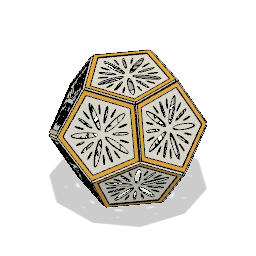
20-Day 14 - Diwali LampShade v2 (Autodesk Fusion 360 design; units mm, degrees)
Autodesk Fusion 360 part; units mm, degrees
(part 1 of 3)
sketch "Sketch1" plane through (0, 0, 0) normal (0, 1, 0) x (1, 0, 0)
  line L0 (-50, 0) -> (-15.4508, -47.5528)
  line L1 (-15.4508, -47.5528) -> (40.4508, -29.3893)
  line L2 (40.4508, -29.3893) -> (40.4508, 29.3893)
  line L3 (40.4508, 29.3893) -> (-15.4508, 47.5528)
  line L4 (-15.4508, 47.5528) -> (-50, 0)
  line L5 (-13.541, -41.675) -> (35.4508, -25.7565)
  line L6 (35.4508, -25.7565) -> (35.4508, 25.7565)
  line L7 (35.4508, 25.7565) -> (-13.541, 41.675)
  line L8 (-13.541, 41.675) -> (-43.8197, 0)
  line L9 (-43.8197, 0) -> (-13.541, -41.675)
  spline S0 degree 5 poles (-5, 0) (-5, 0.1873) (-5.1504, 0.5619) (-5.827, 1.1149) (-7.5942, 1.7986) (-11.0069, 2.4812) (-15.2799, 2.923) (-20, 3.0764) (-24.7201, 2.923) (-28.9931, 2.4812) (-32.4058, 1.7986) (-34.6148, 0.944) (-35.3821, 0) (-34.6148, -0.944) (-32.4058, -1.7986) (-28.9931, -2.4812) (-24.7201, -2.923) (-20, -3.0764) (-15.2799, -2.923) (-11.0069, -2.4812) (-7.5942, -1.7986) (-5.827, -1.1149) (-5.1504, -0.5619) (-5, -0.1873) (-5, 0) knots 0 0 0 0 0 0 0.05 0.1 0.15 0.2 0.25 0.3 0.35 0.4 0.45 0.5 0.55 0.6 0.65 0.7 0.75 0.8 0.85 0.9 0.95 1 1 1 1 1 1
  spline S1 degree 5 poles (-1.5451, -4.7553) (-1.7232, -4.6974) (-2.126, -4.7246) (-2.861, -5.1973) (-4.0573, -6.6667) (-5.7611, -9.7015) (-7.5016, -13.6288) (-9.1062, -18.0705) (-10.4188, -22.607) (-11.3191, -26.8073) (-11.7245, -30.264) (-11.5944, -32.6289) (-10.9337, -33.6504) (-9.7987, -33.2123) (-8.3034, -31.3756) (-6.5996, -28.3408) (-4.8591, -24.4135) (-3.2545, -19.9718) (-1.9418, -15.4352) (-1.0416, -11.2349) (-0.6361, -7.7783) (-0.7403, -5.8864) (-1.0571, -5.0719) (-1.3669, -4.8132) (-1.5451, -4.7553) knots 0 0 0 0 0 0 0.05 0.1 0.15 0.2 0.25 0.3 0.35 0.4 0.45 0.5 0.55 0.6 0.65 0.7 0.75 0.8 0.85 0.9 0.95 1 1 1 1 1 1
  spline S2 degree 5 poles (4.0451, -2.9389) (3.935, -3.0905) (3.8364, -3.4819) (4.0588, -4.327) (5.0866, -5.9189) (7.4464, -8.477) (10.6436, -11.346) (14.3721, -14.2446) (18.281, -16.8949) (21.9975, -19.049) (25.1597, -20.5028) (27.449, -21.1098) (28.6247, -20.7971) (28.5588, -19.5823) (27.2741, -17.5926) (24.9143, -15.0344) (21.7171, -12.1654) (17.9886, -9.2668) (14.0797, -6.6166) (10.3632, -4.4624) (7.201, -3.0086) (5.3695, -2.523) (4.497, -2.5727) (4.1552, -2.7874) (4.0451, -2.9389) knots 0 0 0 0 0 0 0.05 0.1 0.15 0.2 0.25 0.3 0.35 0.4 0.45 0.5 0.55 0.6 0.65 0.7 0.75 0.8 0.85 0.9 0.95 1 1 1 1 1 1
  spline S3 degree 5 poles (4.0451, 2.9389) (4.1552, 2.7874) (4.497, 2.5727) (5.3695, 2.523) (7.201, 3.0086) (10.3632, 4.4624) (14.0797, 6.6166) (17.9886, 9.2668) (21.7171, 12.1654) (24.9143, 15.0344) (27.2741, 17.5926) (28.5588, 19.5823) (28.6247, 20.7971) (27.449, 21.1098) (25.1597, 20.5028) (21.9975, 19.049) (18.281, 16.8949) (14.3721, 14.2446) (10.6436, 11.346) (7.4464, 8.477) (5.0866, 5.9189) (4.0588, 4.327) (3.8364, 3.4819) (3.935, 3.0905) (4.0451, 2.9389) knots 0 0 0 0 0 0 0.05 0.1 0.15 0.2 0.25 0.3 0.35 0.4 0.45 0.5 0.55 0.6 0.65 0.7 0.75 0.8 0.85 0.9 0.95 1 1 1 1 1 1
  spline S4 degree 5 poles (-1.5451, 4.7553) (-1.3669, 4.8132) (-1.0571, 5.0719) (-0.7403, 5.8864) (-0.6361, 7.7783) (-1.0416, 11.2349) (-1.9418, 15.4352) (-3.2545, 19.9718) (-4.8591, 24.4135) (-6.5996, 28.3408) (-8.3034, 31.3756) (-9.7987, 33.2123) (-10.9337, 33.6504) (-11.5944, 32.6289) (-11.7245, 30.264) (-11.3191, 26.8073) (-10.4188, 22.607) (-9.1062, 18.0705) (-7.5016, 13.6288) (-5.7611, 9.7015) (-4.0573, 6.6667) (-2.861, 5.1973) (-2.126, 4.7246) (-1.7232, 4.6974) (-1.5451, 4.7553) knots 0 0 0 0 0 0 0.05 0.1 0.15 0.2 0.25 0.3 0.35 0.4 0.45 0.5 0.55 0.6 0.65 0.7 0.75 0.8 0.85 0.9 0.95 1 1 1 1 1 1
  spline S5 degree 5 poles (-10, 7.2654) (-9.946, 7.3337) (-9.9164, 7.5257) (-10.1101, 7.9769) (-10.8326, 8.8775) (-12.3971, 10.3808) (-14.4507, 12.1067) (-16.7835, 13.883) (-19.1692, 15.538) (-21.3871, 16.9176) (-23.2347, 17.8934) (-24.5416, 18.3712) (-25.1825, 18.2995) (-25.0928, 17.6796) (-24.2842, 16.5762) (-22.8328, 15.1015) (-20.8692, 13.4003) (-18.5684, 11.6352) (-16.1427, 9.973) (-13.8307, 8.571) (-11.8705, 7.5662) (-10.7531, 7.1642) (-10.2405, 7.1161) (-10.054, 7.1972) (-10, 7.2654) knots 0 0 0 0 0 0 0.05 0.1 0.15 0.2 0.25 0.3 0.35 0.4 0.45 0.5 0.55 0.6 0.65 0.7 0.75 0.8 0.85 0.9 0.95 1 1 1 1 1 1
  line L10 (-25, 17.7501) -> (-25, 18.1636)
  spline S6 degree 5 poles (-10, -7.2654) (-10.0482, -7.193) (-10.2217, -7.1055) (-10.7106, -7.1503) (-11.7904, -7.5591) (-13.7037, -8.5825) (-15.9796, -10.0023) (-18.3899, -11.672) (-20.7012, -13.4295) (-22.6985, -15.1125) (-24.1976, -16.5682) (-25.0558, -17.6634) (-25.1857, -18.2951) (-24.5684, -18.4014) (-23.2691, -17.9733) (-21.4181, -17.0487) (-19.1933, -15.7069) (-16.8037, -14.0642) (-14.4732, -12.2708) (-12.4254, -10.5052) (-10.864, -8.9514) (-10.1364, -8.013) (-9.9323, -7.5403) (-9.9518, -7.3379) (-10, -7.2654) knots 0 0 0 0 0 0 0.05 0.1 0.15 0.2 0.25 0.3 0.35 0.4 0.45 0.5 0.55 0.6 0.65 0.7 0.75 0.8 0.85 0.9 0.95 1 1 1 1 1 1
  spline S7 degree 5 poles (3.8197, -11.7557) (3.7358, -11.7792) (3.5991, -11.9171) (3.4905, -12.396) (3.5457, -13.5492) (3.9278, -15.6851) (4.5748, -18.2884) (5.4179, -21.0967) (6.3752, -23.8379) (7.3586, -26.2576) (8.2798, -28.1331) (9.0562, -29.2878) (9.6169, -29.6065) (9.9087, -29.0523) (9.9031, -27.6843) (9.5957, -25.6382) (9.0071, -23.1077) (8.1832, -20.3273) (7.1977, -17.5567) (6.1514, -15.0636) (5.1561, -13.0984) (4.4885, -12.1165) (4.102, -11.7763) (3.9035, -11.7322) (3.8197, -11.7557) knots 0 0 0 0 0 0 0.05 0.1 0.15 0.2 0.25 0.3 0.35 0.4 0.45 0.5 0.55 0.6 0.65 0.7 0.75 0.8 0.85 0.9 0.95 1 1 1 1 1 1
  spline S8 degree 5 poles (12.3607, 0) (12.3571, -0.087) (12.4461, -0.2597) (12.8679, -0.5109) (13.9818, -0.8148) (16.1312, -1.1114) (18.807, -1.3006) (21.7384, -1.3665) (24.6413, -1.3031) (27.2464, -1.1156) (29.3148, -0.819) (30.6529, -0.4374) (31.1293, -0.0027) (30.6923, 0.4461) (29.3895, 0.8635) (27.3486, 1.2034) (24.76, 1.4256) (21.8612, 1.5012) (18.9217, 1.4201) (16.2272, 1.1955) (14.0507, 0.8561) (12.9105, 0.5246) (12.4675, 0.2622) (12.3643, 0.087) (12.3607, 0) knots 0 0 0 0 0 0 0.05 0.1 0.15 0.2 0.25 0.3 0.35 0.4 0.45 0.5 0.55 0.6 0.65 0.7 0.75 0.8 0.85 0.9 0.95 1 1 1 1 1 1
  spline S9 degree 5 poles (3.8197, 11.7557) (3.9013, 11.7254) (4.093, 11.7567) (4.4623, 12.0802) (5.0955, 13.0457) (6.0418, 14.9982) (7.0486, 17.4846) (8.0171, 20.2521) (8.8539, 23.0326) (9.4806, 25.5681) (9.8377, 27.6269) (9.8883, 29.0174) (9.622, 29.6049) (9.0602, 29.328) (8.2607, 28.2179) (7.3067, 26.3819) (6.2955, 23.9887) (5.3278, 21.2551) (4.4965, 18.4344) (3.8775, 15.8024) (3.5277, 13.6276) (3.4906, 12.4407) (3.6033, 11.9383) (3.738, 11.786) (3.8197, 11.7557) knots 0 0 0 0 0 0 0.05 0.1 0.15 0.2 0.25 0.3 0.35 0.4 0.45 0.5 0.55 0.6 0.65 0.7 0.75 0.8 0.85 0.9 0.95 1 1 1 1 1 1
  line L11 (0, 0) -> (32.2957, 0) construction
  line L12 (-20, 1) -> (-20, 3)
  spline S10 degree 5 poles (-20, 6.4984) (-19.9899, 6.5417) (-20.0193, 6.6469) (-20.2127, 6.8586) (-20.7593, 7.2342) (-21.8513, 7.8023) (-23.2443, 8.4014) (-24.806, 8.9632) (-26.3896, 9.4283) (-27.8444, 9.7572) (-29.0275, 9.9285) (-29.8175, 9.9359) (-30.1281, 9.7856) (-29.9216, 9.4946) (-29.2253, 9.0882) (-28.1165, 8.5994) (-26.7091, 8.0666) (-25.1409, 7.5331) (-23.5615, 7.0456) (-22.1199, 6.6533) (-20.9537, 6.4023) (-20.3331, 6.3432) (-20.08, 6.3871) (-20.0101, 6.4551) (-20, 6.4984) knots 0 0 0 0 0 0 0.05 0.1 0.15 0.2 0.25 0.3 0.35 0.4 0.45 0.5 0.55 0.6 0.65 0.7 0.75 0.8 0.85 0.9 0.95 1 1 1 1 1 1
  spline S11 degree 5 poles (-12.3607, 17.013) (-12.3987, 16.99) (-12.5079, 16.9855) (-12.769, 17.104) (-13.2951, 17.5078) (-14.1729, 18.3708) (-15.1731, 19.5105) (-16.19, 20.8221) (-17.1217, 22.1845) (-17.884, 23.4664) (-18.4126, 24.5387) (-18.6637, 25.2878) (-18.6168, 25.6296) (-18.2761, 25.5232) (-17.6745, 24.9865) (-16.867, 24.083) (-15.9253, 22.9091) (-14.9334, 21.5826) (-13.9816, 20.2311) (-13.1631, 18.9813) (-12.564, 17.9497) (-12.316, 17.3778) (-12.2796, 17.1234) (-12.3226, 17.036) (-12.3607, 17.013) knots 0 0 0 0 0 0 0.05 0.1 0.15 0.2 0.25 0.3 0.35 0.4 0.45 0.5 0.55 0.6 0.65 0.7 0.75 0.8 0.85 0.9 0.95 1 1 1 1 1 1
  line L13 (-20.0391, 6.3312) -> (-19.9609, 6.6656)
  line L14 (-12.2137, 17.1018) -> (-12.5076, 16.9242)
  line L15 (-30, 9.7063) -> (-30, 9.7476)
  spline S12 degree 5 poles (-12.3607, -17.013) (-12.3987, -16.99) (-12.5079, -16.9855) (-12.769, -17.104) (-13.2951, -17.5078) (-14.1729, -18.3708) (-15.1731, -19.5105) (-16.19, -20.8221) (-17.1217, -22.1845) (-17.884, -23.4664) (-18.4126, -24.5387) (-18.6637, -25.2878) (-18.6168, -25.6296) (-18.2761, -25.5232) (-17.6745, -24.9865) (-16.867, -24.083) (-15.9253, -22.9091) (-14.9334, -21.5826) (-13.9816, -20.2311) (-13.1631, -18.9813) (-12.564, -17.9497) (-12.316, -17.3778) (-12.2796, -17.1234) (-12.3226, -17.036) (-12.3607, -17.013) knots 0 0 0 0 0 0 0.05 0.1 0.15 0.2 0.25 0.3 0.35 0.4 0.45 0.5 0.55 0.6 0.65 0.7 0.75 0.8 0.85 0.9 0.95 1 1 1 1 1 1
  spline S13 degree 5 poles (-20, -6.4984) (-19.9899, -6.5417) (-20.0193, -6.6469) (-20.2127, -6.8586) (-20.7593, -7.2342) (-21.8513, -7.8023) (-23.2443, -8.4014) (-24.806, -8.9632) (-26.3896, -9.4283) (-27.8444, -9.7572) (-29.0275, -9.9285) (-29.8175, -9.9359) (-30.1281, -9.7856) (-29.9216, -9.4946) (-29.2253, -9.0882) (-28.1165, -8.5994) (-26.7091, -8.0666) (-25.1409, -7.5331) (-23.5615, -7.0456) (-22.1199, -6.6533) (-20.9537, -6.4023) (-20.3331, -6.3432) (-20.08, -6.3871) (-20.0101, -6.4551) (-20, -6.4984) knots 0 0 0 0 0 0 0.05 0.1 0.15 0.2 0.25 0.3 0.35 0.4 0.45 0.5 0.55 0.6 0.65 0.7 0.75 0.8 0.85 0.9 0.95 1 1 1 1 1 1
  spline S14 degree 5 poles (12.3607, -17.013) (12.3271, -17.0421) (12.289, -17.1445) (12.321, -17.4295) (12.5425, -18.0546) (13.092, -19.1561) (13.8668, -20.4596) (14.8, -21.8319) (15.8079, -23.1391) (16.7914, -24.2602) (17.6479, -25.0943) (18.2827, -25.5646) (18.6223, -25.6256) (18.6264, -25.2688) (18.3019, -24.5307) (17.6921, -23.4835) (16.8667, -22.2252) (15.9116, -20.8719) (14.9204, -19.5491) (13.9846, -18.3844) (13.1887, -17.4958) (12.7214, -17.0832) (12.4908, -16.97) (12.3943, -16.9839) (12.3607, -17.013) knots 0 0 0 0 0 0 0.05 0.1 0.15 0.2 0.25 0.3 0.35 0.4 0.45 0.5 0.55 0.6 0.65 0.7 0.75 0.8 0.85 0.9 0.95 1 1 1 1 1 1
  spline S15 degree 5 poles (0, -21.0292) (0.0443, -21.033) (0.1353, -21.0935) (0.2769, -21.3429) (0.4652, -21.9788) (0.668, -23.1929) (0.8073, -24.7028) (0.859, -26.3617) (0.812, -28.0115) (0.6753, -29.4967) (0.4726, -30.6748) (0.2355, -31.4285) (-0.0034, -31.6774) (-0.2164, -31.3911) (-0.3877, -30.6034) (-0.51, -29.3977) (-0.5818, -27.8946) (-0.6046, -26.2383) (-0.5802, -24.5855) (-0.5077, -23.0932) (-0.3861, -21.9065) (-0.2506, -21.2981) (-0.1305, -21.0709) (-0.0443, -21.0255) (0, -21.0292) knots 0 0 0 0 0 0 0.05 0.1 0.15 0.2 0.25 0.3 0.35 0.4 0.45 0.5 0.55 0.6 0.65 0.7 0.75 0.8 0.85 0.9 0.95 1 1 1 1 1 1
  spline S16 degree 5 poles (20, 6.4984) (20.0173, 6.4574) (20.1029, 6.3896) (20.3838, 6.332) (21.0468, 6.3494) (22.2642, 6.5317) (23.7433, 6.8658) (25.3369, 7.3292) (26.8915, 7.8838) (28.2617, 8.4728) (29.3196, 9.0296) (29.9631, 9.488) (30.126, 9.7921) (29.7879, 9.9062) (28.9857, 9.8257) (27.8013, 9.5694) (26.3495, 9.1732) (24.7673, 8.6831) (23.2029, 8.1491) (21.8061, 7.6191) (20.715, 7.1367) (20.1783, 6.8198) (19.9993, 6.6354) (19.9827, 6.5394) (20, 6.4984) knots 0 0 0 0 0 0 0.05 0.1 0.15 0.2 0.25 0.3 0.35 0.4 0.45 0.5 0.55 0.6 0.65 0.7 0.75 0.8 0.85 0.9 0.95 1 1 1 1 1 1
  spline S17 degree 5 poles (20, -6.4984) (20.0173, -6.4574) (20.1029, -6.3896) (20.3838, -6.332) (21.0468, -6.3494) (22.2642, -6.5317) (23.7433, -6.8658) (25.3369, -7.3292) (26.8915, -7.8838) (28.2617, -8.4728) (29.3196, -9.0296) (29.9631, -9.488) (30.126, -9.7921) (29.7879, -9.9062) (28.9857, -9.8257) (27.8013, -9.5694) (26.3495, -9.1732) (24.7673, -8.6831) (23.2029, -8.1491) (21.8061, -7.6191) (20.715, -7.1367) (20.1783, -6.8198) (19.9993, -6.6354) (19.9827, -6.5394) (20, -6.4984) knots 0 0 0 0 0 0 0.05 0.1 0.15 0.2 0.25 0.3 0.35 0.4 0.45 0.5 0.55 0.6 0.65 0.7 0.75 0.8 0.85 0.9 0.95 1 1 1 1 1 1
  spline S18 degree 5 poles (0, 21.0292) (0.0443, 21.033) (0.1353, 21.0935) (0.2769, 21.3429) (0.4652, 21.9788) (0.668, 23.1929) (0.8073, 24.7028) (0.859, 26.3617) (0.812, 28.0115) (0.6753, 29.4967) (0.4726, 30.6748) (0.2355, 31.4285) (-0.0034, 31.6774) (-0.2164, 31.3911) (-0.3877, 30.6034) (-0.51, 29.3977) (-0.5818, 27.8946) (-0.6046, 26.2383) (-0.5802, 24.5855) (-0.5077, 23.0932) (-0.3861, 21.9065) (-0.2506, 21.2981) (-0.1305, 21.0709) (-0.0443, 21.0255) (0, 21.0292) knots 0 0 0 0 0 0 0.05 0.1 0.15 0.2 0.25 0.3 0.35 0.4 0.45 0.5 0.55 0.6 0.65 0.7 0.75 0.8 0.85 0.9 0.95 1 1 1 1 1 1
  spline S19 degree 5 poles (12.3607, 17.013) (12.3271, 17.0421) (12.289, 17.1445) (12.321, 17.4295) (12.5425, 18.0546) (13.092, 19.1561) (13.8668, 20.4596) (14.8, 21.8319) (15.8079, 23.1391) (16.7914, 24.2602) (17.6479, 25.0943) (18.2827, 25.5646) (18.6223, 25.6256) (18.6264, 25.2688) (18.3019, 24.5307) (17.6921, 23.4835) (16.8667, 22.2252) (15.9116, 20.8719) (14.9204, 19.5491) (13.9846, 18.3844) (13.1887, 17.4958) (12.7214, 17.0832) (12.4908, 16.97) (12.3943, 16.9839) (12.3607, 17.013) knots 0 0 0 0 0 0 0.05 0.1 0.15 0.2 0.25 0.3 0.35 0.4 0.45 0.5 0.55 0.6 0.65 0.7 0.75 0.8 0.85 0.9 0.95 1 1 1 1 1 1
  line L16 (-30, 9.7476) -> (-30.715, 9.9799)
  line L17 (6.4347, -102.4282) -> (6.459, -102.4616)
  line L18 (12.5094, -93.8428) -> (12.7692, -94.0674)
  spline S20 degree 5 poles (5, -70.4437) (4.9827, -70.4847) (4.8971, -70.5525) (4.6162, -70.6101) (3.9532, -70.5927) (2.7358, -70.4104) (1.2567, -70.0763) (-0.3369, -69.6129) (-1.8915, -69.0583) (-3.2617, -68.4693) (-4.3196, -67.9125) (-4.9631, -67.4541) (-5.126, -67.15) (-4.7879, -67.0358) (-3.9857, -67.1164) (-2.8013, -67.3727) (-1.3495, -67.7689) (0.2327, -68.259) (1.7971, -68.7929) (3.1939, -69.323) (4.285, -69.8054) (4.8217, -70.1223) (5.0007, -70.3067) (5.0173, -70.4027) (5, -70.4437) knots 0 0 0 0 0 0 0.05 0.1 0.15 0.2 0.25 0.3 0.35 0.4 0.45 0.5 0.55 0.6 0.65 0.7 0.75 0.8 0.85 0.9 0.95 1 1 1 1 1 1
  line L19 (-12.2076, -17.1055) -> (-12.5137, -16.9205)
  line L20 (5.0695, -70.2789) -> (4.9305, -70.6085)
  spline S21 degree 5 poles (12.6393, -76.9421) (12.6429, -77.0291) (12.5539, -77.2018) (12.1321, -77.453) (11.0182, -77.7569) (8.8688, -78.0535) (6.193, -78.2426) (3.2616, -78.3086) (0.3587, -78.2452) (-2.2464, -78.0577) (-4.3148, -77.7611) (-5.6529, -77.3795) (-6.1293, -76.9448) (-5.6923, -76.496) (-4.3895, -76.0786) (-2.3486, -75.7387) (0.24, -75.5165) (3.1388, -75.4409) (6.0783, -75.522) (8.7728, -75.7466) (10.9493, -76.086) (12.0895, -76.4175) (12.5325, -76.6799) (12.6357, -76.8551) (12.6393, -76.9421) knots 0 0 0 0 0 0 0.05 0.1 0.15 0.2 0.25 0.3 0.35 0.4 0.45 0.5 0.55 0.6 0.65 0.7 0.75 0.8 0.85 0.9 0.95 1 1 1 1 1 1
  line L21 (-9.8099, -7.5511) -> (-10.1901, -6.9798)
  line L22 (12.6252, -76.5992) -> (12.6534, -77.285)
  spline S22 degree 5 poles (26.5451, -72.1868) (26.3669, -72.1289) (26.0571, -71.8701) (25.7403, -71.0557) (25.6361, -69.1638) (26.0416, -65.7072) (26.9418, -61.5068) (28.2545, -56.9703) (29.8591, -52.5286) (31.5996, -48.6013) (33.3034, -45.5665) (34.7987, -43.7298) (35.9337, -43.2917) (36.5944, -44.3132) (36.7245, -46.6781) (36.3191, -50.1348) (35.4188, -54.3351) (34.1062, -58.8716) (32.5016, -63.3133) (30.7611, -67.2406) (29.0573, -70.2754) (27.861, -71.7448) (27.126, -72.2174) (26.7232, -72.2447) (26.5451, -72.1868) knots 0 0 0 0 0 0 0.05 0.1 0.15 0.2 0.25 0.3 0.35 0.4 0.45 0.5 0.55 0.6 0.65 0.7 0.75 0.8 0.85 0.9 0.95 1 1 1 1 1 1
  line L23 (4.487, -2.3307) -> (3.6032, -3.5472)
  line L24 (27.2601, -72.4191) -> (25.8301, -71.9545)
  spline S23 degree 5 poles (21.1803, -65.1864) (21.0987, -65.2167) (20.907, -65.1854) (20.5377, -64.8619) (19.9045, -63.8964) (18.9582, -61.9439) (17.9514, -59.4575) (16.9829, -56.6899) (16.1461, -53.9095) (15.5194, -51.3739) (15.1623, -49.3152) (15.1117, -47.9247) (15.378, -47.3372) (15.9398, -47.6141) (16.7393, -48.7242) (17.6933, -50.5602) (18.7045, -52.9534) (19.6722, -55.687) (20.5035, -58.5077) (21.1225, -61.1397) (21.4723, -63.3145) (21.5094, -64.5014) (21.3967, -65.0038) (21.262, -65.1561) (21.1803, -65.1864) knots 0 0 0 0 0 0 0.05 0.1 0.15 0.2 0.25 0.3 0.35 0.4 0.45 0.5 0.55 0.6 0.65 0.7 0.75 0.8 0.85 0.9 0.95 1 1 1 1 1 1
  line L25 (4.1359, -11.6671) -> (3.5034, -11.8443)
  line L26 (21.4883, -65.0722) -> (20.8724, -65.3006)
  spline S24 degree 5 poles (5, -83.4405) (4.9827, -83.3995) (4.8971, -83.3317) (4.6162, -83.2741) (3.9532, -83.2915) (2.7358, -83.4737) (1.2567, -83.8079) (-0.3369, -84.2713) (-1.8915, -84.8259) (-3.2617, -85.4149) (-4.3196, -85.9716) (-4.9631, -86.4301) (-5.126, -86.7342) (-4.7879, -86.8483) (-3.9857, -86.7678) (-2.8013, -86.5115) (-1.3495, -86.1153) (0.2327, -85.6252) (1.7971, -85.0912) (3.1939, -84.5612) (4.285, -84.0788) (4.8217, -83.7619) (5.0007, -83.5775) (5.0173, -83.4815) (5, -83.4405) knots 0 0 0 0 0 0 0.05 0.1 0.15 0.2 0.25 0.3 0.35 0.4 0.45 0.5 0.55 0.6 0.65 0.7 0.75 0.8 0.85 0.9 0.95 1 1 1 1 1 1
  line L27 (-20.0391, -6.3312) -> (-19.9609, -6.6656)
  line L28 (5.0667, -83.5987) -> (4.9333, -83.2822)
  line L29 (-15.4508, -106.3314) -> (-15.4508, -47.5528)
  line L30 (-10.4508, -102.6986) -> (-10.4508, -51.1855)
  line L31 (38.541, -118.6171) -> (-10.4508, -102.6986)
  line L32 (68.8197, -76.9421) -> (38.541, -118.6171)
  spline S25 degree 5 poles (37.3607, -93.9551) (37.3987, -93.9321) (37.5079, -93.9276) (37.769, -94.0461) (38.2951, -94.4499) (39.1729, -95.3129) (40.1731, -96.4526) (41.19, -97.7642) (42.1217, -99.1266) (42.884, -100.4085) (43.4126, -101.4808) (43.6637, -102.2299) (43.6168, -102.5716) (43.2761, -102.4653) (42.6745, -101.9286) (41.867, -101.0251) (40.9253, -99.8512) (39.9334, -98.5247) (38.9816, -97.1732) (38.1631, -95.9234) (37.564, -94.8918) (37.316, -94.3199) (37.2796, -94.0655) (37.3226, -93.9781) (37.3607, -93.9551) knots 0 0 0 0 0 0 0.05 0.1 0.15 0.2 0.25 0.3 0.35 0.4 0.45 0.5 0.55 0.6 0.65 0.7 0.75 0.8 0.85 0.9 0.95 1 1 1 1 1 1
  line L33 (-0.1589, 21.0158) -> (0.1589, 21.0427)
  line L34 (37.2242, -94.0376) -> (37.4971, -93.8726)
  line L35 (6.459, -102.4616) -> (6.0171, -103.0699)
  line L36 (9.4074, -89.5068) -> (10.583, -91.1248)
  line L37 (25, -76.9421) -> (51.1278, -57.9592) construction
  spline S26 degree 5 poles (35, -69.6767) (34.946, -69.6084) (34.9164, -69.4164) (35.1101, -68.9652) (35.8326, -68.0646) (37.3971, -66.5613) (39.4507, -64.8354) (41.7835, -63.0591) (44.1692, -61.4041) (46.3871, -60.0245) (48.2347, -59.0487) (49.5416, -58.5709) (50.1825, -58.6426) (50.0928, -59.2625) (49.2842, -60.3659) (47.8328, -61.8406) (45.8692, -63.5418) (43.5684, -65.3069) (41.1427, -66.9691) (38.8307, -68.3711) (36.8705, -69.3759) (35.7531, -69.7779) (35.2405, -69.826) (35.054, -69.7449) (35, -69.6767) knots 0 0 0 0 0 0 0.05 0.1 0.15 0.2 0.25 0.3 0.35 0.4 0.45 0.5 0.55 0.6 0.65 0.7 0.75 0.8 0.85 0.9 0.95 1 1 1 1 1 1
  line L38 (12.3731, 0.3028) -> (12.3482, -0.3028)
  line L39 (35.1881, -69.9144) -> (34.8119, -69.439)
  line L40 (40.4508, -124.4949) -> (-15.4508, -106.3314)
  line L41 (75, -76.9421) -> (40.4508, -124.4949)
  spline S27 degree 5 poles (30, -76.9421) (30, -76.7548) (30.1504, -76.3801) (30.827, -75.8271) (32.5942, -75.1435) (36.0069, -74.4609) (40.2799, -74.0191) (45, -73.8657) (49.7201, -74.0191) (53.9931, -74.4609) (57.4058, -75.1435) (59.6148, -75.9981) (60.3821, -76.9421) (59.6148, -77.8861) (57.4058, -78.7407) (53.9931, -79.4233) (49.7201, -79.865) (45, -80.0185) (40.2799, -79.865) (36.0069, -79.4233) (32.5942, -78.7407) (30.827, -78.057) (30.1504, -77.504) (30, -77.1294) (30, -76.9421) knots 0 0 0 0 0 0 0.05 0.1 0.15 0.2 0.25 0.3 0.35 0.4 0.45 0.5 0.55 0.6 0.65 0.7 0.75 0.8 0.85 0.9 0.95 1 1 1 1 1 1
  line L42 (3.6032, 3.5472) -> (4.487, 2.3307)
  line L43 (30, -77.6939) -> (30, -76.1903)
  spline S28 degree 5 poles (21.1803, -88.6978) (21.2642, -88.7213) (21.4009, -88.8592) (21.5095, -89.338) (21.4543, -90.4913) (21.0722, -92.6272) (20.4252, -95.2305) (19.5821, -98.0388) (18.6248, -100.78) (17.6414, -103.1997) (16.7202, -105.0752) (15.9438, -106.2299) (15.3831, -106.5486) (15.0913, -105.9944) (15.0969, -104.6264) (15.4043, -102.5803) (15.9929, -100.0497) (16.8168, -97.2694) (17.8023, -94.4988) (18.8486, -92.0057) (19.8439, -90.0405) (20.5115, -89.0585) (20.898, -88.7184) (21.0965, -88.6743) (21.1803, -88.6978) knots 0 0 0 0 0 0 0.05 0.1 0.15 0.2 0.25 0.3 0.35 0.4 0.45 0.5 0.55 0.6 0.65 0.7 0.75 0.8 0.85 0.9 0.95 1 1 1 1 1 1
  line L44 (-10.2129, 6.9964) -> (-9.7871, 7.5345)
  line L45 (20.85, -88.6053) -> (21.5107, -88.7903)
  spline S29 degree 5 poles (26.5451, -81.6974) (26.7232, -81.6395) (27.126, -81.6667) (27.861, -82.1394) (29.0573, -83.6088) (30.7611, -86.6436) (32.5016, -90.5709) (34.1062, -95.0126) (35.4188, -99.5491) (36.3191, -103.7494) (36.7245, -107.2061) (36.5944, -109.571) (35.9337, -110.5925) (34.7987, -110.1544) (33.3034, -108.3177) (31.5996, -105.2829) (29.8591, -101.3556) (28.2545, -96.9139) (26.9418, -92.3773) (26.0416, -88.177) (25.6361, -84.7204) (25.7403, -82.8285) (26.0571, -82.014) (26.3669, -81.7553) (26.5451, -81.6974) knots 0 0 0 0 0 0 0.05 0.1 0.15 0.2 0.25 0.3 0.35 0.4 0.45 0.5 0.55 0.6 0.65 0.7 0.75 0.8 0.85 0.9 0.95 1 1 1 1 1 1
  line L46 (-2.2225, 4.5352) -> (-0.8676, 4.9754)
  line L47 (25.8676, -81.9175) -> (27.2225, -81.4773)
  spline S30 degree 5 poles (25, -97.9713) (24.9557, -97.9751) (24.8647, -98.0356) (24.7231, -98.285) (24.5348, -98.9209) (24.332, -100.135) (24.1927, -101.6449) (24.141, -103.3037) (24.188, -104.9536) (24.3247, -106.4388) (24.5274, -107.6169) (24.7645, -108.3706) (25.0034, -108.6195) (25.2164, -108.3332) (25.3877, -107.5454) (25.51, -106.3398) (25.5818, -104.8366) (25.6046, -103.1804) (25.5802, -101.5276) (25.5077, -100.0353) (25.3861, -98.8486) (25.2506, -98.2402) (25.1305, -98.013) (25.0443, -97.9676) (25, -97.9713) knots 0 0 0 0 0 0 0.05 0.1 0.15 0.2 0.25 0.3 0.35 0.4 0.45 0.5 0.55 0.6 0.65 0.7 0.75 0.8 0.85 0.9 0.95 1 1 1 1 1 1
  line L48 (25.1711, -97.9568) -> (24.8289, -97.9859)
  spline S31 degree 5 poles (25, -55.9128) (24.9557, -55.9091) (24.8647, -55.8486) (24.7231, -55.5992) (24.5348, -54.9633) (24.332, -53.7492) (24.1927, -52.2393) (24.141, -50.5804) (24.188, -48.9306) (24.3247, -47.4454) (24.5274, -46.2672) (24.7645, -45.5136) (25.0034, -45.2647) (25.2164, -45.5509) (25.3877, -46.3387) (25.51, -47.5444) (25.5818, -49.0475) (25.6046, -50.7038) (25.5802, -52.3565) (25.5077, -53.8488) (25.3861, -55.0356) (25.2506, -55.644) (25.1305, -55.8712) (25.0443, -55.9166) (25, -55.9128) knots 0 0 0 0 0 0 0.05 0.1 0.15 0.2 0.25 0.3 0.35 0.4 0.45 0.5 0.55 0.6 0.65 0.7 0.75 0.8 0.85 0.9 0.95 1 1 1 1 1 1
  line L49 (12.4959, -16.8961) -> (12.2255, -17.1299)
  line L50 (25.1781, -55.928) -> (24.8219, -55.8977)
  spline S32 degree 5 poles (20.9549, -79.881) (21.065, -80.0326) (21.1636, -80.424) (20.9412, -81.2691) (19.9134, -82.8609) (17.5536, -85.4191) (14.3564, -88.2881) (10.6279, -91.1867) (6.719, -93.8369) (3.0025, -95.9911) (-0.1597, -97.4449) (-2.449, -98.0519) (-3.6247, -97.7392) (-3.5588, -96.5244) (-2.2741, -94.5346) (0.0857, -91.9765) (3.2829, -89.1075) (7.0114, -86.2089) (10.9203, -83.5586) (14.6368, -81.4045) (17.799, -79.9507) (19.6305, -79.4651) (20.503, -79.5148) (20.8448, -79.7295) (20.9549, -79.881) knots 0 0 0 0 0 0 0.05 0.1 0.15 0.2 0.25 0.3 0.35 0.4 0.45 0.5 0.55 0.6 0.65 0.7 0.75 0.8 0.85 0.9 0.95 1 1 1 1 1 1
  line L51 (-5, -0.6433) -> (-5, 0.6433)
  line L52 (20.5768, -79.3606) -> (21.333, -80.4015)
  line L53 (38.541, -35.2671) -> (68.8197, -76.9421)
  line L54 (40.4508, -29.3893) -> (75, -76.9421)
  line L55 (-10.4508, -51.1855) -> (38.541, -35.2671)
  spline S33 degree 5 poles (12.6393, -59.9291) (12.6729, -59.9) (12.711, -59.7976) (12.679, -59.5126) (12.4575, -58.8875) (11.908, -57.786) (11.1332, -56.4825) (10.2, -55.1101) (9.1921, -53.803) (8.2086, -52.6818) (7.3521, -51.8478) (6.7173, -51.3775) (6.3777, -51.3165) (6.3736, -51.6733) (6.6981, -52.4113) (7.3079, -53.4586) (8.1333, -54.7169) (9.0884, -56.0702) (10.0796, -57.393) (11.0154, -58.5577) (11.8113, -59.4463) (12.2786, -59.8588) (12.5092, -59.9721) (12.6057, -59.9582) (12.6393, -59.9291) knots 0 0 0 0 0 0 0.05 0.1 0.15 0.2 0.25 0.3 0.35 0.4 0.45 0.5 0.55 0.6 0.65 0.7 0.75 0.8 0.85 0.9 0.95 1 1 1 1 1 1
  line L56 (-0.1589, -21.0158) -> (0.1589, -21.0427)
  line L57 (12.5187, -60.0334) -> (12.7599, -59.8248)
  spline S34 degree 5 poles (20.9549, -74.0032) (20.8448, -74.1547) (20.503, -74.3694) (19.6305, -74.4191) (17.799, -73.9335) (14.6368, -72.4797) (10.9203, -70.3255) (7.0114, -67.6753) (3.2829, -64.7767) (0.0857, -61.9077) (-2.2741, -59.3495) (-3.5588, -57.3598) (-3.6247, -56.145) (-2.449, -55.8323) (-0.1597, -56.4393) (3.0025, -57.8931) (6.719, -60.0472) (10.6279, -62.6975) (14.3564, -65.5961) (17.5536, -68.4651) (19.9134, -71.0232) (20.9412, -72.615) (21.1636, -73.4602) (21.065, -73.8516) (20.9549, -74.0032) knots 0 0 0 0 0 0 0.05 0.1 0.15 0.2 0.25 0.3 0.35 0.4 0.45 0.5 0.55 0.6 0.65 0.7 0.75 0.8 0.85 0.9 0.95 1 1 1 1 1 1
  line L58 (-0.8676, -4.9754) -> (-2.2225, -4.5352)
  line L59 (21.3736, -73.4269) -> (20.5362, -74.5794)
  spline S35 degree 5 poles (37.3607, -59.9291) (37.3987, -59.9521) (37.5079, -59.9566) (37.769, -59.8381) (38.2951, -59.4343) (39.1729, -58.5713) (40.1731, -57.4316) (41.19, -56.12) (42.1217, -54.7575) (42.884, -53.4756) (43.4126, -52.4034) (43.6637, -51.6543) (43.6168, -51.3125) (43.2761, -51.4189) (42.6745, -51.9556) (41.867, -52.8591) (40.9253, -54.033) (39.9334, -55.3595) (38.9816, -56.7109) (38.1631, -57.9608) (37.564, -58.9924) (37.316, -59.5643) (37.2796, -59.8186) (37.3226, -59.9061) (37.3607, -59.9291) knots 0 0 0 0 0 0 0.05 0.1 0.15 0.2 0.25 0.3 0.35 0.4 0.45 0.5 0.55 0.6 0.65 0.7 0.75 0.8 0.85 0.9 0.95 1 1 1 1 1 1
  line L60 (19.9334, -6.6564) -> (20.0666, -6.3404)
  line L61 (37.2139, -59.8404) -> (37.5074, -60.0178)
  spline S36 degree 5 poles (35, -84.2075) (35.0482, -84.1351) (35.2217, -84.0476) (35.7106, -84.0923) (36.7904, -84.5012) (38.7037, -85.5246) (40.9796, -86.9444) (43.3899, -88.6141) (45.7012, -90.3716) (47.6985, -92.0546) (49.1976, -93.5103) (50.0558, -94.6055) (50.1857, -95.2372) (49.5684, -95.3435) (48.2691, -94.9154) (46.4181, -93.9907) (44.1933, -92.649) (41.8037, -91.0062) (39.4732, -89.2129) (37.4254, -87.4473) (35.864, -85.8935) (35.1364, -84.9551) (34.9323, -84.4824) (34.9518, -84.28) (35, -84.2075) knots 0 0 0 0 0 0 0.05 0.1 0.15 0.2 0.25 0.3 0.35 0.4 0.45 0.5 0.55 0.6 0.65 0.7 0.75 0.8 0.85 0.9 0.95 1 1 1 1 1 1
  line L62 (3.5119, 11.8699) -> (4.1274, 11.6415)
  line L63 (34.8181, -84.4808) -> (35.1819, -83.9343)
  line L64 (15.2078, -105.9969) -> (15.4508, -106.3314)
  spline S37 degree 5 poles (45, -83.4405) (44.9899, -83.4838) (45.0193, -83.589) (45.2127, -83.8007) (45.7593, -84.1763) (46.8513, -84.7444) (48.2443, -85.3435) (49.806, -85.9053) (51.3896, -86.3704) (52.8444, -86.6993) (54.0275, -86.8706) (54.8175, -86.878) (55.1281, -86.7277) (54.9216, -86.4366) (54.2253, -86.0303) (53.1165, -85.5415) (51.7091, -85.0087) (50.1409, -84.4752) (48.5615, -83.9876) (47.1199, -83.5954) (45.9537, -83.3444) (45.3331, -83.2853) (45.08, -83.3292) (45.0101, -83.3972) (45, -83.4405) knots 0 0 0 0 0 0 0.05 0.1 0.15 0.2 0.25 0.3 0.35 0.4 0.45 0.5 0.55 0.6 0.65 0.7 0.75 0.8 0.85 0.9 0.95 1 1 1 1 1 1
  line L65 (12.4959, 16.8961) -> (12.2255, 17.1299)
  line L66 (45.0407, -83.2664) -> (44.9593, -83.6146)
  spline S38 degree 5 poles (12.6393, -93.9551) (12.6729, -93.9842) (12.711, -94.0866) (12.679, -94.3716) (12.4575, -94.9967) (11.908, -96.0982) (11.1332, -97.4016) (10.2, -98.774) (9.1921, -100.0812) (8.2086, -101.2023) (7.3521, -102.0364) (6.7173, -102.5067) (6.3777, -102.5677) (6.3736, -102.2108) (6.6981, -101.4728) (7.3079, -100.4256) (8.1333, -99.1673) (9.0884, -97.814) (10.0796, -96.4912) (11.0154, -95.3265) (11.8113, -94.4379) (12.2786, -94.0253) (12.5092, -93.9121) (12.6057, -93.926) (12.6393, -93.9551) knots 0 0 0 0 0 0 0.05 0.1 0.15 0.2 0.25 0.3 0.35 0.4 0.45 0.5 0.55 0.6 0.65 0.7 0.75 0.8 0.85 0.9 0.95 1 1 1 1 1 1
  line L67 (12.5094, -93.8428) -> (12.7692, -94.0674)
  spline S39 degree 5 poles (45, -70.4437) (44.9899, -70.4004) (45.0193, -70.2952) (45.2127, -70.0835) (45.7593, -69.7079) (46.8513, -69.1398) (48.2443, -68.5407) (49.806, -67.9789) (51.3896, -67.5138) (52.8444, -67.1849) (54.0275, -67.0135) (54.8175, -67.0062) (55.1281, -67.1564) (54.9216, -67.4475) (54.2253, -67.8539) (53.1165, -68.3427) (51.7091, -68.8755) (50.1409, -69.409) (48.5615, -69.8965) (47.1199, -70.2888) (45.9537, -70.5398) (45.3331, -70.5989) (45.08, -70.5549) (45.0101, -70.487) (45, -70.4437) knots 0 0 0 0 0 0 0.05 0.1 0.15 0.2 0.25 0.3 0.35 0.4 0.45 0.5 0.55 0.6 0.65 0.7 0.75 0.8 0.85 0.9 0.95 1 1 1 1 1 1
  line L68 (19.9334, 6.6564) -> (20.0666, 6.3404)
  line L69 (45.039, -70.6107) -> (44.961, -70.2767)
  line L70 (25.1711, -97.9568) -> (24.8289, -97.9859)
  line L71 (-45.4146, -53.896) -> (-45.4871, -54.2065)
  line L72 (-65.28, -68.5676) -> (-65.6217, -68.5966)
  line L73 (-60.4508, -48.2651) -> (-60.4508, -46.8405)
  line L74 (-55.6328, -55.0917) -> (-55.2689, -54.5448)
  line L75 (-53.2432, -64.6583) -> (-52.9372, -64.4734)
  spline S40 degree 5 poles (-65.4508, -68.5821) (-65.4952, -68.5858) (-65.5861, -68.6463) (-65.7277, -68.8957) (-65.916, -69.5316) (-66.1189, -70.7457) (-66.2582, -72.2557) (-66.3099, -73.9145) (-66.2628, -75.5644) (-66.1261, -77.0495) (-65.9235, -78.2277) (-65.6864, -78.9813) (-65.4475, -79.2302) (-65.2344, -78.944) (-65.0631, -78.1562) (-64.9409, -76.9505) (-64.8691, -75.4474) (-64.8463, -73.7911) (-64.8707, -72.1384) (-64.9431, -70.6461) (-65.0647, -69.4594) (-65.2003, -68.8509) (-65.3203, -68.6237) (-65.4065, -68.5783) (-65.4508, -68.5821) knots 0 0 0 0 0 0 0.05 0.1 0.15 0.2 0.25 0.3 0.35 0.4 0.45 0.5 0.55 0.6 0.65 0.7 0.75 0.8 0.85 0.9 0.95 1 1 1 1 1 1
  line L76 (-65.28, -68.5676) -> (-65.6217, -68.5966)
  spline S41 degree 5 poles (-45.4508, -41.0544) (-45.461, -41.0111) (-45.4316, -40.9059) (-45.2381, -40.6942) (-44.6916, -40.3186) (-43.5996, -39.7505) (-42.2065, -39.1514) (-40.6449, -38.5896) (-39.0612, -38.1246) (-37.6065, -37.7956) (-36.4234, -37.6243) (-35.6333, -37.6169) (-35.3228, -37.7672) (-35.5292, -38.0583) (-36.2255, -38.4646) (-37.3344, -38.9534) (-38.7418, -39.4862) (-40.3099, -40.0197) (-41.8893, -40.5073) (-43.331, -40.8995) (-44.4972, -41.1505) (-45.1177, -41.2097) (-45.3709, -41.1657) (-45.4407, -41.0977) (-45.4508, -41.0544) knots 0 0 0 0 0 0 0.05 0.1 0.15 0.2 0.25 0.3 0.35 0.4 0.45 0.5 0.55 0.6 0.65 0.7 0.75 0.8 0.85 0.9 0.95 1 1 1 1 1 1
  line L77 (-45.4102, -41.2286) -> (-45.4915, -40.8803)
  line L78 (-53.2371, -30.451) -> (-52.9432, -30.6286)
  spline S42 degree 5 poles (-53.0902, -30.5398) (-53.0521, -30.5628) (-52.943, -30.5674) (-52.6818, -30.4488) (-52.1557, -30.0451) (-51.278, -29.1821) (-50.2777, -28.0423) (-49.2609, -26.7307) (-48.3292, -25.3683) (-47.5668, -24.0864) (-47.0383, -23.0142) (-46.7871, -22.265) (-46.8341, -21.9233) (-47.1747, -22.0296) (-47.7763, -22.5663) (-48.5839, -23.4698) (-49.5255, -24.6437) (-50.5175, -25.9702) (-51.4692, -27.3217) (-52.2878, -28.5716) (-52.8869, -29.6031) (-53.1349, -30.175) (-53.1713, -30.4294) (-53.1282, -30.5168) (-53.0902, -30.5398) knots 0 0 0 0 0 0 0.05 0.1 0.15 0.2 0.25 0.3 0.35 0.4 0.45 0.5 0.55 0.6 0.65 0.7 0.75 0.8 0.85 0.9 0.95 1 1 1 1 1 1
  line L79 (-53.2371, -30.451) -> (-52.9432, -30.6286)
  line L80 (-55.2379, -40.5565) -> (-55.6638, -40.0183)
  spline S43 degree 5 poles (-45.4508, -54.0512) (-45.461, -54.0945) (-45.4316, -54.1997) (-45.2381, -54.4115) (-44.6916, -54.787) (-43.5996, -55.3552) (-42.2065, -55.9542) (-40.6449, -56.516) (-39.0612, -56.9811) (-37.6065, -57.31) (-36.4234, -57.4814) (-35.6333, -57.4888) (-35.3228, -57.3385) (-35.5292, -57.0474) (-36.2255, -56.641) (-37.3344, -56.1522) (-38.7418, -55.6194) (-40.3099, -55.0859) (-41.8893, -54.5984) (-43.331, -54.2061) (-44.4972, -53.9551) (-45.1177, -53.896) (-45.3709, -53.94) (-45.4407, -54.0079) (-45.4508, -54.0512) knots 0 0 0 0 0 0 0.05 0.1 0.15 0.2 0.25 0.3 0.35 0.4 0.45 0.5 0.55 0.6 0.65 0.7 0.75 0.8 0.85 0.9 0.95 1 1 1 1 1 1
  line L81 (-45.4146, -53.896) -> (-45.4871, -54.2065)
  line L82 (-85.3889, -40.9075) -> (-85.5128, -41.2013)
  spline S44 degree 5 poles (-65.4508, -26.5236) (-65.4952, -26.5198) (-65.5861, -26.4593) (-65.7277, -26.2099) (-65.916, -25.5741) (-66.1189, -24.36) (-66.2582, -22.85) (-66.3099, -21.1912) (-66.2628, -19.5413) (-66.1261, -18.0561) (-65.9235, -16.878) (-65.6864, -16.1243) (-65.4475, -15.8754) (-65.2344, -16.1617) (-65.0631, -16.9495) (-64.9409, -18.1551) (-64.8691, -19.6583) (-64.8463, -21.3145) (-64.8707, -22.9673) (-64.9431, -24.4596) (-65.0647, -25.6463) (-65.2003, -26.2547) (-65.3203, -26.4819) (-65.4065, -26.5273) (-65.4508, -26.5236) knots 0 0 0 0 0 0 0.05 0.1 0.15 0.2 0.25 0.3 0.35 0.4 0.45 0.5 0.55 0.6 0.65 0.7 0.75 0.8 0.85 0.9 0.95 1 1 1 1 1 1
  line L83 (-65.2797, -26.5381) -> (-65.622, -26.5091)
  spline S45 degree 5 poles (-69.2705, -59.3085) (-69.1867, -59.332) (-69.0499, -59.47) (-68.9414, -59.9488) (-68.9965, -61.1021) (-69.3786, -63.2379) (-70.0256, -65.8412) (-70.8688, -68.6495) (-71.8261, -71.3908) (-72.8095, -73.8104) (-73.7307, -75.6859) (-74.5071, -76.8406) (-75.0678, -77.1593) (-75.3596, -76.6051) (-75.3539, -75.2371) (-75.0465, -73.191) (-74.4579, -70.6605) (-73.634, -67.8801) (-72.6486, -65.1096) (-71.6023, -62.6164) (-70.607, -60.6513) (-69.9393, -59.6693) (-69.5529, -59.3291) (-69.3543, -59.2851) (-69.2705, -59.3085) knots 0 0 0 0 0 0 0.05 0.1 0.15 0.2 0.25 0.3 0.35 0.4 0.45 0.5 0.55 0.6 0.65 0.7 0.75 0.8 0.85 0.9 0.95 1 1 1 1 1 1
  line L84 (-69.5624, -59.2268) -> (-68.9786, -59.3903)
  line L85 (-68.9489, -35.6778) -> (-69.5922, -35.9164)
  spline S46 degree 5 poles (-77.8115, -47.5528) (-77.808, -47.6398) (-77.8969, -47.8125) (-78.3187, -48.0637) (-79.4326, -48.3676) (-81.582, -48.6642) (-84.2579, -48.8534) (-87.1892, -48.9193) (-90.0921, -48.856) (-92.6973, -48.6684) (-94.7656, -48.3718) (-96.1037, -47.9902) (-96.5801, -47.5555) (-96.1432, -47.1067) (-94.8404, -46.6894) (-92.7994, -46.3494) (-90.2109, -46.1273) (-87.312, -46.0516) (-84.3725, -46.1327) (-81.678, -46.3574) (-79.5015, -46.6967) (-78.3613, -47.0282) (-77.9183, -47.2907) (-77.8151, -47.4659) (-77.8115, -47.5528) knots 0 0 0 0 0 0 0.05 0.1 0.15 0.2 0.25 0.3 0.35 0.4 0.45 0.5 0.55 0.6 0.65 0.7 0.75 0.8 0.85 0.9 0.95 1 1 1 1 1 1
  line L86 (-77.825, -47.2249) -> (-77.7981, -47.8808)
  spline S47 degree 5 poles (-69.2705, -35.7971) (-69.3521, -35.8274) (-69.5439, -35.7962) (-69.9131, -35.4726) (-70.5464, -34.5072) (-71.4927, -32.5546) (-72.4994, -30.0682) (-73.468, -27.3007) (-74.3048, -24.5203) (-74.9314, -21.9847) (-75.2885, -19.9259) (-75.3391, -18.5354) (-75.0729, -17.948) (-74.511, -18.2249) (-73.7115, -19.3349) (-72.7575, -21.1709) (-71.7463, -23.5641) (-70.7786, -26.2977) (-69.9473, -29.1184) (-69.3284, -31.7504) (-68.9785, -33.9253) (-68.9415, -35.1122) (-69.0542, -35.6145) (-69.1889, -35.7668) (-69.2705, -35.7971) knots 0 0 0 0 0 0 0.05 0.1 0.15 0.2 0.25 0.3 0.35 0.4 0.45 0.5 0.55 0.6 0.65 0.7 0.75 0.8 0.85 0.9 0.95 1 1 1 1 1 1
  line L87 (-68.9489, -35.6778) -> (-69.5922, -35.9164)
  line L88 (-69.9378, -49.8835) -> (-69.054, -51.1)
  line L89 (-77.9412, -64.4537) -> (-77.6818, -64.678)
  line L90 (-77.825, -47.2249) -> (-77.7981, -47.8808)
  line L91 (-69.5624, -59.2268) -> (-68.9786, -59.3903)
  spline S48 degree 5 poles (-77.8115, -64.5658) (-77.7779, -64.5949) (-77.7398, -64.6973) (-77.7719, -64.9823) (-77.9933, -65.6074) (-78.5428, -66.7089) (-79.3177, -68.0124) (-80.2509, -69.3848) (-81.2587, -70.6919) (-82.2423, -71.8131) (-83.0987, -72.6471) (-83.7335, -73.1175) (-84.0731, -73.1784) (-84.0772, -72.8216) (-83.7527, -72.0836) (-83.143, -71.0363) (-82.3175, -69.778) (-81.3624, -68.4247) (-80.3712, -67.1019) (-79.4355, -65.9372) (-78.6395, -65.0486) (-78.1723, -64.6361) (-77.9416, -64.5228) (-77.8452, -64.5368) (-77.8115, -64.5658) knots 0 0 0 0 0 0 0.05 0.1 0.15 0.2 0.25 0.3 0.35 0.4 0.45 0.5 0.55 0.6 0.65 0.7 0.75 0.8 0.85 0.9 0.95 1 1 1 1 1 1
  line L92 (-77.9412, -64.4537) -> (-77.6818, -64.678)
  spline S49 degree 5 poles (-85.4509, -54.0512) (-85.4681, -54.0103) (-85.5538, -53.9424) (-85.8347, -53.8848) (-86.4976, -53.9022) (-87.715, -54.0845) (-89.1941, -54.4186) (-90.7877, -54.882) (-92.3423, -55.4366) (-93.7126, -56.0256) (-94.7704, -56.5824) (-95.4139, -57.0408) (-95.5768, -57.3449) (-95.2387, -57.4591) (-94.4366, -57.3785) (-93.2522, -57.1222) (-91.8004, -56.726) (-90.2181, -56.2359) (-88.6538, -55.702) (-87.2569, -55.1719) (-86.1659, -54.6895) (-85.6291, -54.3726) (-85.4501, -54.1882) (-85.4336, -54.0922) (-85.4509, -54.0512) knots 0 0 0 0 0 0 0.05 0.1 0.15 0.2 0.25 0.3 0.35 0.4 0.45 0.5 0.55 0.6 0.65 0.7 0.75 0.8 0.85 0.9 0.95 1 1 1 1 1 1
  line L93 (-85.3814, -54.2159) -> (-85.5203, -53.8865)
  spline S50 degree 5 poles (-63.9058, -42.7975) (-64.0839, -42.7397) (-64.3937, -42.4809) (-64.7106, -41.6665) (-64.8147, -39.7745) (-64.4092, -36.3179) (-63.509, -32.1176) (-62.1964, -27.581) (-60.5918, -23.1393) (-58.8512, -19.2121) (-57.1475, -16.1773) (-55.6521, -14.3405) (-54.5172, -13.9024) (-53.8565, -14.9239) (-53.7263, -17.2889) (-54.1318, -20.7455) (-55.032, -24.9458) (-56.3447, -29.4824) (-57.9492, -33.9241) (-59.6898, -37.8513) (-61.3935, -40.8861) (-62.5898, -42.3555) (-63.3249, -42.8282) (-63.7276, -42.8554) (-63.9058, -42.7975) knots 0 0 0 0 0 0 0.05 0.1 0.15 0.2 0.25 0.3 0.35 0.4 0.45 0.5 0.55 0.6 0.65 0.7 0.75 0.8 0.85 0.9 0.95 1 1 1 1 1 1
  line L94 (-63.2939, -42.9963) -> (-64.5176, -42.5988)
  line L95 (-85.3814, -54.2159) -> (-85.5203, -53.8865)
  line L96 (-74.6068, -18.2913) -> (-75, -18.1635)
  spline S51 degree 5 poles (-85.4509, -41.0544) (-85.4681, -41.0954) (-85.5538, -41.1632) (-85.8347, -41.2208) (-86.4976, -41.2034) (-87.715, -41.0212) (-89.1941, -40.687) (-90.7877, -40.2236) (-92.3423, -39.669) (-93.7126, -39.08) (-94.7704, -38.5233) (-95.4139, -38.0649) (-95.5768, -37.7607) (-95.2387, -37.6466) (-94.4366, -37.7271) (-93.2522, -37.9834) (-91.8004, -38.3796) (-90.2181, -38.8698) (-88.6538, -39.4037) (-87.2569, -39.9337) (-86.1659, -40.4161) (-85.6291, -40.733) (-85.4501, -40.9174) (-85.4336, -41.0135) (-85.4509, -41.0544) knots 0 0 0 0 0 0 0.05 0.1 0.15 0.2 0.25 0.3 0.35 0.4 0.45 0.5 0.55 0.6 0.65 0.7 0.75 0.8 0.85 0.9 0.95 1 1 1 1 1 1
  line L97 (-85.3889, -40.9075) -> (-85.5128, -41.2013)
  line L98 (-60.2216, -28.2227) -> (-62.1237, -27.6046)
  line L99 (-65.4508, -47.5528) -> (-75.4308, -78.2679) construction
  spline S52 degree 5 poles (-69.4959, -44.6139) (-69.606, -44.7654) (-69.9479, -44.9801) (-70.8204, -45.0298) (-72.6519, -44.5442) (-75.814, -43.0904) (-79.5306, -40.9363) (-83.4395, -38.286) (-87.1679, -35.3874) (-90.3651, -32.5184) (-92.7249, -29.9603) (-94.0097, -27.9705) (-94.0756, -26.7557) (-92.8999, -26.443) (-90.6105, -27.0501) (-87.4483, -28.5038) (-83.7318, -30.658) (-79.8229, -33.3082) (-76.0944, -36.2068) (-72.8973, -39.0758) (-70.5375, -41.634) (-69.5097, -43.2258) (-69.2873, -44.0709) (-69.3858, -44.4624) (-69.4959, -44.6139) knots 0 0 0 0 0 0 0.05 0.1 0.15 0.2 0.25 0.3 0.35 0.4 0.45 0.5 0.55 0.6 0.65 0.7 0.75 0.8 0.85 0.9 0.95 1 1 1 1 1 1
  line L100 (-69.0772, -44.0376) -> (-69.9146, -45.1902)
  line L101 (-69.0772, -44.0376) -> (-69.9146, -45.1902)
  line L102 (-65.2797, -26.5381) -> (-65.622, -26.5091)
  line L103 (-64.6208, -52.5404) -> (-63.1907, -52.0758)
  line L104 (-65.4508, -16.009) -> (-65.4508, -15.2571)
  line L105 (-65.4116, -16.0217) -> (-65.4508, -16.009)
  spline S53 degree 5 poles (-77.8115, -30.5398) (-77.7779, -30.5107) (-77.7398, -30.4083) (-77.7719, -30.1233) (-77.9933, -29.4982) (-78.5428, -28.3967) (-79.3177, -27.0933) (-80.2509, -25.7209) (-81.2587, -24.4138) (-82.2423, -23.2926) (-83.0987, -22.4585) (-83.7335, -21.9882) (-84.0731, -21.9272) (-84.0772, -22.2841) (-83.7527, -23.0221) (-83.143, -24.0693) (-82.3175, -25.3276) (-81.3624, -26.681) (-80.3712, -28.0037) (-79.4355, -29.1684) (-78.6395, -30.057) (-78.1723, -30.4696) (-77.9416, -30.5828) (-77.8452, -30.5689) (-77.8115, -30.5398) knots 0 0 0 0 0 0 0.05 0.1 0.15 0.2 0.25 0.3 0.35 0.4 0.45 0.5 0.55 0.6 0.65 0.7 0.75 0.8 0.85 0.9 0.95 1 1 1 1 1 1
  line L106 (-77.9414, -30.6521) -> (-77.6816, -30.4275)
  spline S54 degree 5 poles (-69.4959, -50.4918) (-69.3858, -50.6433) (-69.2873, -51.0348) (-69.5097, -51.8799) (-70.5375, -53.4717) (-72.8973, -56.0298) (-76.0944, -58.8988) (-79.8229, -61.7974) (-83.7318, -64.4477) (-87.4483, -66.6018) (-90.6105, -68.0556) (-92.8999, -68.6626) (-94.0756, -68.3499) (-94.0097, -67.1351) (-92.7249, -65.1454) (-90.3651, -62.5872) (-87.1679, -59.7182) (-83.4395, -56.8197) (-79.5306, -54.1694) (-75.814, -52.0152) (-72.6519, -50.5615) (-70.8204, -50.0759) (-69.9479, -50.1255) (-69.606, -50.3402) (-69.4959, -50.4918) knots 0 0 0 0 0 0 0.05 0.1 0.15 0.2 0.25 0.3 0.35 0.4 0.45 0.5 0.55 0.6 0.65 0.7 0.75 0.8 0.85 0.9 0.95 1 1 1 1 1 1
  line L107 (-69.9378, -49.8835) -> (-69.054, -51.1)
  line L108 (-63.2939, -42.9963) -> (-64.5176, -42.5988)
  line L109 (-77.9414, -30.6521) -> (-77.6816, -30.4275)
  spline S55 degree 5 poles (-53.0902, -64.5658) (-53.0521, -64.5428) (-52.943, -64.5383) (-52.6818, -64.6568) (-52.1557, -65.0606) (-51.278, -65.9236) (-50.2777, -67.0633) (-49.2609, -68.3749) (-48.3292, -69.7374) (-47.5668, -71.0193) (-47.0383, -72.0915) (-46.7871, -72.8406) (-46.8341, -73.1824) (-47.1747, -73.076) (-47.7763, -72.5394) (-48.5839, -71.6358) (-49.5255, -70.4619) (-50.5175, -69.1354) (-51.4692, -67.784) (-52.2878, -66.5341) (-52.8869, -65.5025) (-53.1349, -64.9306) (-53.1713, -64.6763) (-53.1282, -64.5888) (-53.0902, -64.5658) knots 0 0 0 0 0 0 0.05 0.1 0.15 0.2 0.25 0.3 0.35 0.4 0.45 0.5 0.55 0.6 0.65 0.7 0.75 0.8 0.85 0.9 0.95 1 1 1 1 1 1
  line L110 (-53.2432, -64.6583) -> (-52.9372, -64.4734)
  spline S56 degree 5 poles (-60.4508, -47.5528) (-60.4508, -47.3655) (-60.3005, -46.9909) (-59.6238, -46.4379) (-57.8567, -45.7542) (-54.4439, -45.0717) (-50.171, -44.6299) (-45.4508, -44.4764) (-40.7307, -44.6299) (-36.4578, -45.0717) (-33.045, -45.7542) (-30.8361, -46.6088) (-30.0687, -47.5528) (-30.8361, -48.4969) (-33.045, -49.3514) (-36.4578, -50.034) (-40.7307, -50.4758) (-45.4508, -50.6293) (-50.171, -50.4758) (-54.4439, -50.034) (-57.8567, -49.3514) (-59.6238, -48.6678) (-60.3005, -48.1148) (-60.4508, -47.7401) (-60.4508, -47.5528) knots 0 0 0 0 0 0 0.05 0.1 0.15 0.2 0.25 0.3 0.35 0.4 0.45 0.5 0.55 0.6 0.65 0.7 0.75 0.8 0.85 0.9 0.95 1 1 1 1 1 1
  line L111 (-60.4508, -48.2651) -> (-60.4508, -46.8405)
  spline S57 degree 5 poles (-55.4508, -40.2874) (-55.5049, -40.2191) (-55.5344, -40.0271) (-55.3408, -39.576) (-54.6183, -38.6754) (-53.0537, -37.172) (-51.0001, -35.4462) (-48.6673, -33.6698) (-46.2816, -32.0148) (-44.0638, -30.6353) (-42.2161, -29.6594) (-40.9093, -29.1816) (-40.2683, -29.2533) (-40.358, -29.8732) (-41.1667, -30.9767) (-42.618, -32.4513) (-44.5816, -34.1526) (-46.8824, -35.9176) (-49.3082, -37.5798) (-51.6201, -38.9819) (-53.5804, -39.9867) (-54.6977, -40.3887) (-55.2103, -40.4367) (-55.3968, -40.3557) (-55.4508, -40.2874) knots 0 0 0 0 0 0 0.05 0.1 0.15 0.2 0.25 0.3 0.35 0.4 0.45 0.5 0.55 0.6 0.65 0.7 0.75 0.8 0.85 0.9 0.95 1 1 1 1 1 1
  line L112 (-55.2379, -40.5565) -> (-55.6638, -40.0183)
  line L113 (-45.4102, -41.2286) -> (-45.4915, -40.8803)
  spline S58 degree 5 poles (-55.4508, -54.8183) (-55.4026, -54.7458) (-55.2291, -54.6584) (-54.7402, -54.7031) (-53.6604, -55.1119) (-51.7472, -56.1353) (-49.4712, -57.5551) (-47.0609, -59.2248) (-44.7497, -60.9823) (-42.7523, -62.6653) (-41.2533, -64.121) (-40.3951, -65.2162) (-40.2652, -65.848) (-40.8825, -65.9542) (-42.1818, -65.5261) (-44.0327, -64.6015) (-46.2575, -63.2597) (-48.6472, -61.617) (-50.9776, -59.8236) (-53.0254, -58.0581) (-54.5868, -56.5042) (-55.3144, -55.5658) (-55.5185, -55.0931) (-55.4991, -54.8907) (-55.4508, -54.8183) knots 0 0 0 0 0 0 0.05 0.1 0.15 0.2 0.25 0.3 0.35 0.4 0.45 0.5 0.55 0.6 0.65 0.7 0.75 0.8 0.85 0.9 0.95 1 1 1 1 1 1
  line L114 (-55.6328, -55.0917) -> (-55.2689, -54.5448)
  spline S59 degree 5 poles (-63.9058, -52.3081) (-63.7276, -52.2502) (-63.3249, -52.2775) (-62.5898, -52.7501) (-61.3935, -54.2195) (-59.6898, -57.2543) (-57.9492, -61.1816) (-56.3447, -65.6233) (-55.032, -70.1598) (-54.1318, -74.3602) (-53.7263, -77.8168) (-53.8565, -80.1817) (-54.5172, -81.2032) (-55.6521, -80.7651) (-57.1475, -78.9284) (-58.8512, -75.8936) (-60.5918, -71.9663) (-62.1964, -67.5246) (-63.509, -62.9881) (-64.4092, -58.7878) (-64.8147, -55.3311) (-64.7106, -53.4392) (-64.3937, -52.6248) (-64.0839, -52.366) (-63.9058, -52.3081) knots 0 0 0 0 0 0 0.05 0.1 0.15 0.2 0.25 0.3 0.35 0.4 0.45 0.5 0.55 0.6 0.65 0.7 0.75 0.8 0.85 0.9 0.95 1 1 1 1 1 1
  line L115 (-64.6208, -52.5404) -> (-63.1907, -52.0758)
  line L116 (-105.9017, -18.1636) -> (-50, 0)
  line L117 (-100.9017, -21.7963) -> (-51.9098, -5.8779)
  line L118 (-100.9017, -73.3094) -> (-100.9017, -21.7963)
  line L119 (-105.9017, -76.9421) -> (-105.9017, -18.1636)
  line L120 (-51.9098, -89.2278) -> (-100.9017, -73.3094)
  line L121 (-50, -95.1057) -> (-105.9017, -76.9421)
  line L122 (-21.6312, -47.5528) -> (-51.9098, -89.2278)
  line L123 (-51.9098, -5.8779) -> (-21.6312, -47.5528)
  line L124 (-15.4508, -47.5528) -> (-50, -95.1057)
  line L125 (-46.9491, 22.0205) -> (-46.9098, 22.0333)
  line L126 (-21.6312, 47.5528) -> (-51.9098, 5.8779)
  line L127 (-68.9863, 59.4139) -> (-69.5547, 59.2031)
  line L128 (-55.2472, 54.5608) -> (-55.6545, 55.0757)
  line L129 (-60.4508, 46.8405) -> (-60.4508, 48.2651)
  line L130 (-45.4118, 41.2217) -> (-45.4899, 40.8872)
  spline S60 degree 5 poles (-55.4508, 54.8183) (-55.5049, 54.8865) (-55.5344, 55.0785) (-55.3408, 55.5297) (-54.6183, 56.4303) (-53.0537, 57.9336) (-51.0001, 59.6595) (-48.6673, 61.4358) (-46.2816, 63.0909) (-44.0638, 64.4704) (-42.2161, 65.4462) (-40.9093, 65.924) (-40.2683, 65.8523) (-40.358, 65.2324) (-41.1667, 64.129) (-42.618, 62.6543) (-44.5816, 60.9531) (-46.8824, 59.188) (-49.3082, 57.5258) (-51.6201, 56.1238) (-53.5804, 55.119) (-54.6977, 54.717) (-55.2103, 54.6689) (-55.3968, 54.75) (-55.4508, 54.8183) knots 0 0 0 0 0 0 0.05 0.1 0.15 0.2 0.25 0.3 0.35 0.4 0.45 0.5 0.55 0.6 0.65 0.7 0.75 0.8 0.85 0.9 0.95 1 1 1 1 1 1
  line L131 (-55.2472, 54.5608) -> (-55.6545, 55.0757)
  line L132 (-46.9098, 22.0333) -> (-46.4679, 21.4251)
  spline S61 degree 5 poles (-45.4508, 54.0512) (-45.461, 54.0945) (-45.4316, 54.1997) (-45.2381, 54.4115) (-44.6916, 54.787) (-43.5996, 55.3552) (-42.2065, 55.9542) (-40.6449, 56.516) (-39.0612, 56.9811) (-37.6065, 57.31) (-36.4234, 57.4814) (-35.6333, 57.4888) (-35.3228, 57.3385) (-35.5292, 57.0474) (-36.2255, 56.641) (-37.3344, 56.1522) (-38.7418, 55.6194) (-40.3099, 55.0859) (-41.8893, 54.5984) (-43.331, 54.2061) (-44.4972, 53.9551) (-45.1177, 53.896) (-45.3709, 53.94) (-45.4407, 54.0079) (-45.4508, 54.0512) knots 0 0 0 0 0 0 0.05 0.1 0.15 0.2 0.25 0.3 0.35 0.4 0.45 0.5 0.55 0.6 0.65 0.7 0.75 0.8 0.85 0.9 0.95 1 1 1 1 1 1
  line L133 (-45.4146, 53.896) -> (-45.4871, 54.2065)
  line L134 (-63.1907, 52.0758) -> (-64.6208, 52.5404)
  line L135 (-50, 0) -> (-105.9017, 18.1636)
  line L136 (-105.9017, 76.9421) -> (-50, 95.1057)
  line L137 (-58.3195, 28.8407) -> (-56.4173, 29.4587)
  line L138 (-50, 95.1057) -> (-15.4508, 47.5528)
  line L139 (-100.9017, 73.3094) -> (-51.9098, 89.2278)
  spline S62 degree 5 poles (-53.0902, 64.5658) (-53.0521, 64.5428) (-52.943, 64.5383) (-52.6818, 64.6568) (-52.1557, 65.0606) (-51.278, 65.9236) (-50.2777, 67.0633) (-49.2609, 68.3749) (-48.3292, 69.7374) (-47.5668, 71.0193) (-47.0383, 72.0915) (-46.7871, 72.8406) (-46.8341, 73.1824) (-47.1747, 73.076) (-47.7763, 72.5394) (-48.5839, 71.6358) (-49.5255, 70.4619) (-50.5175, 69.1354) (-51.4692, 67.784) (-52.2878, 66.5341) (-52.8869, 65.5025) (-53.1349, 64.9306) (-53.1713, 64.6763) (-53.1282, 64.5888) (-53.0902, 64.5658) knots 0 0 0 0 0 0 0.05 0.1 0.15 0.2 0.25 0.3 0.35 0.4 0.45 0.5 0.55 0.6 0.65 0.7 0.75 0.8 0.85 0.9 0.95 1 1 1 1 1 1
  line L140 (-53.2432, 64.6583) -> (-52.9372, 64.4734)
  spline S63 degree 5 poles (-65.4508, 68.5821) (-65.4952, 68.5858) (-65.5861, 68.6463) (-65.7277, 68.8957) (-65.916, 69.5316) (-66.1189, 70.7457) (-66.2582, 72.2557) (-66.3099, 73.9145) (-66.2628, 75.5644) (-66.1261, 77.0495) (-65.9235, 78.2277) (-65.6864, 78.9813) (-65.4475, 79.2302) (-65.2344, 78.944) (-65.0631, 78.1562) (-64.9409, 76.9505) (-64.8691, 75.4474) (-64.8463, 73.7911) (-64.8707, 72.1384) (-64.9431, 70.6461) (-65.0647, 69.4594) (-65.2003, 68.8509) (-65.3203, 68.6237) (-65.4065, 68.5783) (-65.4508, 68.5821) knots 0 0 0 0 0 0 0.05 0.1 0.15 0.2 0.25 0.3 0.35 0.4 0.45 0.5 0.55 0.6 0.65 0.7 0.75 0.8 0.85 0.9 0.95 1 1 1 1 1 1
  line L141 (-65.28, 68.5676) -> (-65.6217, 68.5966)
  spline S64 degree 5 poles (-77.8115, 64.5658) (-77.7779, 64.5949) (-77.7398, 64.6973) (-77.7719, 64.9823) (-77.9933, 65.6074) (-78.5428, 66.7089) (-79.3177, 68.0124) (-80.2509, 69.3848) (-81.2587, 70.6919) (-82.2423, 71.8131) (-83.0987, 72.6471) (-83.7335, 73.1175) (-84.0731, 73.1784) (-84.0772, 72.8216) (-83.7527, 72.0836) (-83.143, 71.0363) (-82.3175, 69.778) (-81.3624, 68.4247) (-80.3712, 67.1019) (-79.4355, 65.9372) (-78.6395, 65.0486) (-78.1723, 64.6361) (-77.9416, 64.5228) (-77.8452, 64.5368) (-77.8115, 64.5658) knots 0 0 0 0 0 0 0.05 0.1 0.15 0.2 0.25 0.3 0.35 0.4 0.45 0.5 0.55 0.6 0.65 0.7 0.75 0.8 0.85 0.9 0.95 1 1 1 1 1 1
  line L142 (-77.9412, 64.4537) -> (-77.6818, 64.678)
  spline S65 degree 5 poles (-85.4509, 41.0544) (-85.4681, 41.0954) (-85.5538, 41.1632) (-85.8347, 41.2208) (-86.4976, 41.2034) (-87.715, 41.0212) (-89.1941, 40.687) (-90.7877, 40.2236) (-92.3423, 39.669) (-93.7126, 39.08) (-94.7704, 38.5233) (-95.4139, 38.0649) (-95.5768, 37.7607) (-95.2387, 37.6466) (-94.4366, 37.7271) (-93.2522, 37.9834) (-91.8004, 38.3796) (-90.2181, 38.8698) (-88.6538, 39.4037) (-87.2569, 39.9337) (-86.1659, 40.4161) (-85.6291, 40.733) (-85.4501, 40.9174) (-85.4336, 41.0135) (-85.4509, 41.0544) knots 0 0 0 0 0 0 0.05 0.1 0.15 0.2 0.25 0.3 0.35 0.4 0.45 0.5 0.55 0.6 0.65 0.7 0.75 0.8 0.85 0.9 0.95 1 1 1 1 1 1
  line L143 (-85.3889, 40.9075) -> (-85.5128, 41.2013)